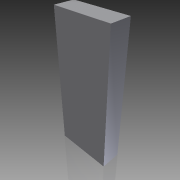
# Autodesk Inventor part: HK 20A BEC
Saved by Autodesk Inventor 2012 (Build 160160000, 160)
## iProperties
Created: 2013-03-10
Part Number: HK 20A BEC
Material: Default
Document SubType Name: Modeling
Designer: fixer
Density: 1 g/cm^3
Mass: 13.4898 g
Surface Area: 45.6128 cm^2
Volume: 13.4898 cm^3
Author: fixer
Autodesk Inventor part; units mm, degrees
ref_plane "YZ Plane" through (0, 0, 0) normal (1, 0, 0) x (0, 1, 0)
ref_plane "XZ Plane" through (0, 0, 0) normal (0, 1, 0) x (-1, 0, 0)
ref_plane "XY Plane" through (0, 0, 0) normal (0, 0, 1) x (1, 0, 0)
sketch "Sketch1" plane through (0, 0, 0) normal (0, 0, 1) x (1, 0, 0)
  line L0 (68.6266, -121.8287) -> (43.7346, -121.8287)
  line L1 (43.7346, -121.8287) -> (43.7346, -60.8687)
  line L2 (43.7346, -60.8687) -> (68.6266, -60.8687)
  line L3 (68.6266, -60.8687) -> (68.6266, -121.8287)
  point P0 (0, 0)
  dimension "d0" = 24.892
  dimension "d1" = 60.96
  constraints: 8 end point, 2 parallel, 1 horizontal, 1 perpendicular
  measures "d0" distance of L1.end L2.end
  measures "d1" distance of L0.end L1.end
extrude "Extrusion1" add sketch "Sketch1" along normal blind 8.89
body "Solid1"
